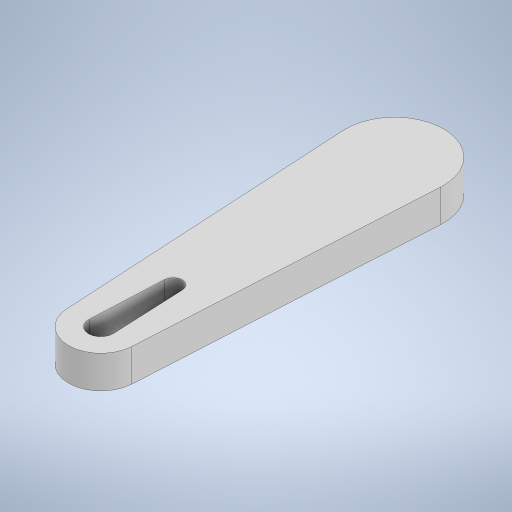
# Autodesk Inventor part: Brazo
Saved by Autodesk Inventor 2024 (Build 280153000, 153)
## iProperties
Created: 2024-04-28
Part Number: Brazo
Material: Generic
Document SubType Name: Modeling
Designer: samue
Density: 1 g/cm^3
Appearance: Default
Author: samue
Autodesk Inventor part; units mm, degrees
ref_plane "YZ Plane" through (0, 0, 0) normal (1, 0, 0) x (0, 1, 0)
ref_plane "XZ Plane" through (0, 0, 0) normal (0, 1, 0) x (-1, 0, 0)
ref_plane "XY Plane" through (0, 0, 0) normal (0, 0, 1) x (1, 0, 0)
sketch "Sketch1" plane through (0, 0, 0) normal (0, 1, 0) x (-1, 0, 0)
  circle A0 centre (-0.0087, 99.7911) radius 10
  circle A1 centre (-0.0022, 9.7911) radius 15
  line L0 (9.9759, 100.3474) -> (14.9746, 10.6255)
  line L1 (-9.9933, 100.346) -> (-14.9791, 10.6234)
  point P0 (0, 0)
  dimension "d0" = 20
  dimension "d1" = 30
  dimension "d2" = 90
  constraints: 4 end point, 4 point on circle, 4 tangent, 2 centre point
  measures "d0" diameter of A0
  measures "d1" diameter of A1
  measures "d2" distance of A1.centre A0.centre
extrude "Extrusion1" add sketch "Sketch1" against normal blind 10
sketch "Sketch2" plane through (0, 0, 0) normal (0, 1, 0) x (1, 0, 0)
  arc A0 (-10.9717, -47.1362) -> (-10.974, -54.1073) centre (-11.2006, -50.6217) ccw
  arc A1 (4.9583, -53.0718) -> (4.96, -48.1823) centre (4.7994, -50.627) ccw
  circle A2 centre (-11.2006, -50.6217) radius 3.5005
  line L0 (-11.2006, -47.1212) -> (4.96, -48.1823)
  line L1 (4.9583, -53.0718) -> (-10.974, -54.1073)
  circle A3 centre (-11.2006, -50.6217) radius 2.5
  circle A4 centre (-11.2006, -50.6217) radius 2.5
  circle A5 centre (0, -99.8683) radius 3.75
  circle A6 centre (0, -77.6683) radius 2.75
  line L2 (2.7472, -77.5444) -> (3.7462, -99.6993)
  line L3 (-3.7462, -99.6993) -> (-2.7472, -77.5444)
  point P0 (0, 0)
  dimension "d5" = 4.9
  dimension "d6" = 16
  dimension "d7" = 7.5
  dimension "d8" = 5.5
  dimension "d9" = 22.2
  constraints: 8 end point, 8 point on circle, 8 tangent, 6 centre point, 2 coincident, 1 point on line, 1 vertical alignment, 2 other
  measures "d5" diameter of A1
  measures "d6" distance of A1.centre point (-11.201, -50.622)
  measures "d7" diameter of A5
  measures "d8" diameter of A6
  measures "d9" distance of A5.centre A6.centre
extrude "Extrusion2" cut sketch "Sketch2" against normal blind 8.5 contours A5 | A5 L3 A6 L2 | A6
sketch "Sketch3" plane through (0, -8.5, 0) normal (0, 1, 0) x (1, 0, 0)
  arc A0 (-3.7462, -99.6993) -> (3.7462, -99.6993) centre (0, -99.8683) ccw projected
  circle A1 centre (0, -99.8683) radius 3.65
  point P0 (0, 0)
  dimension "d12" = 7.3
  constraints: 1 centre point, 1 coincident
  measures "d12" diameter of A1
extrude "Extrusion3" cut sketch "Sketch3" against normal blind 8.5
body "Solid1"
